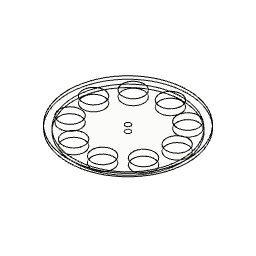
source lid v1 (Autodesk Fusion 360 archive; units mm, degrees)
design "source lid" references "source baseplate sketch", "Global Parameters"
Autodesk Fusion 360 part; units mm, degrees
derive "DerivedContext1" from "assembly of apparatus v94"
derive "Derived from Global Parameters v5" from "Global Parameters v5"
derive "Sketch1" from "source baseplate sketch v14"
sketch "sketch 190" plane through (0, 0, 0) normal (0, 0, 1) x (1, 0, 0)
  line L0 (0, 0) -> (0, 71) construction
  circle A0 centre (0, 71) radius 18
  circle A1 centre (0, 71) radius 19
  circle A2 centre (-45.6379, 54.3892) radius 18
  line L1 (0, 0) -> (-45.6379, 54.3892) construction
  circle A3 centre (-45.6379, 54.3892) radius 19
  circle A4 centre (-69.9214, 12.329) radius 18
  line L2 (0, 0) -> (-69.9214, 12.329) construction
  circle A5 centre (-69.9214, 12.329) radius 19
  circle A6 centre (-61.4878, -35.5) radius 18
  line L3 (0, 0) -> (-61.4878, -35.5) construction
  circle A7 centre (-61.4878, -35.5) radius 19
  circle A8 centre (-24.2834, -66.7182) radius 18
  line L4 (0, 0) -> (-24.2834, -66.7182) construction
  circle A9 centre (-24.2834, -66.7182) radius 19
  circle A10 centre (24.2834, -66.7182) radius 18
  line L5 (0, 0) -> (24.2834, -66.7182) construction
  circle A11 centre (24.2834, -66.7182) radius 19
  circle A12 centre (61.4878, -35.5) radius 18
  line L6 (0, 0) -> (61.4878, -35.5) construction
  circle A13 centre (61.4878, -35.5) radius 19
  circle A14 centre (0, 0) radius 90
  circle A15 centre (0, 0) radius 100
  circle A16 centre (69.9214, 12.329) radius 18
  line L7 (0, 0) -> (69.9214, 12.329) construction
  circle A17 centre (69.9214, 12.329) radius 19
  circle A18 centre (45.6379, 54.3892) radius 18
  line L8 (0, 0) -> (45.6379, 54.3892) construction
  circle A19 centre (45.6379, 54.3892) radius 19
extrude "Extrude1" add sketch "sketch 190" along normal blind 10 contours A0 | A1 | A3 | A5 | A7 | A9 | A11 | A13 | A17 | A19 | A14 | A2 | A4 | A6 | A8 | A10 | A12 | A15 | A16 | A18
extrude "Extrude2" cut sketch "sketch 190" along normal blind 5 contours A8 | A15
extrude "Extrude3" cut sketch "sketch 190" along normal blind 10 contours A0 | A2 | A4 | A6 | A8 | A10 | A12 | A16 | A18
sketch "Sketch1" plane through (0, 0, 10) normal (0, 0, 1) x (-1, 0, 0)
  circle A0 centre (45.6379, -54.3892) radius 18
  circle A1 centre (24.2834, 66.7182) radius 18
  circle A2 centre (0, -71) radius 18
  circle A3 centre (69.9214, -12.329) radius 18
  circle A4 centre (-24.2834, 66.7182) radius 18
  circle A5 centre (-61.4878, 35.5) radius 18
  circle A6 centre (61.4878, 35.5) radius 18
  circle A7 centre (0, 0) radius 100
  circle A8 centre (0, 0) radius 4
  spline S0 degree 11 poles (-4, -0.0001) (-4, -1.7137) (-3.1926, -3.4272) (-1.5768, -4.7182) (0.5947, -5.1627) (2.8314, -4.5085) (4.5073, -2.8299) (5.1631, -0.5961) (4.718, 1.5774) (3.4272, 3.1924) (1.7136, 3.9999) (0, 3.9999) knots 0 0 0 0 0 0 0 0 0 0 0 0 4.945362 4.945362 4.945362 4.945362 4.945362 4.945362 4.945362 4.945362 4.945362 4.945362 4.945362 4.945362
  circle A9 centre (0, 0) radius 4.5
  circle A10 centre (-69.9214, -12.329) radius 18
  circle A11 centre (-45.6379, -54.3892) radius 18
  dimension "d8" = 0.5
  constraint coincident A7.centre A8.centre
  constraint coincident A8 S0.start
extrude "Extrude4" cut sketch "Sketch1" against normal through all contours A8 S0 | A9
equation "pmma_thickness_Ref = 10 mm" comment "The thickness of the Perspex (Poly Methyl Meth Acrylaat) plate"
equation "d2 = pmma_thickness_Ref"
equation "d4 = pmma_thickness_Ref / 2"
equation "d6 = pmma_thickness_Ref"
equation "rotate_motor_Ref = 117 deg"
